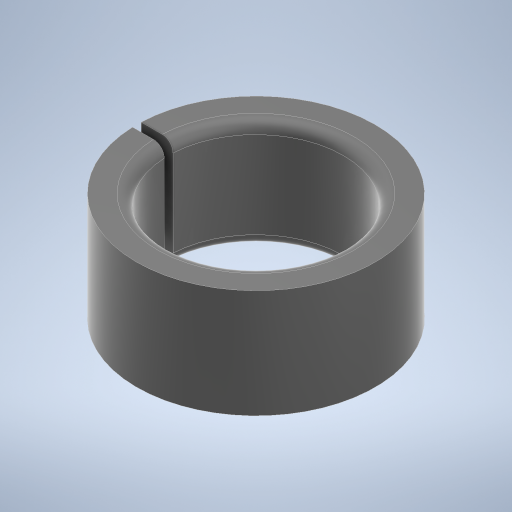
# Autodesk Inventor part: fittingRing
Saved by Autodesk Inventor 2023 (Build 270158000, 158)
## iProperties
Created: 2023-06-24
Part Number: fittingRing
Material: Пластик ПАЭК
Document SubType Name: Modeling
Designer: khrip
Density: 1.32 g/cm^3
Appearance: Гладкая — черная
Author: khrip
Autodesk Inventor part; units mm, degrees
ref_plane "YZ Plane" through (0, 0, 0) normal (1, 0, 0) x (0, 1, 0)
ref_plane "XZ Plane" through (0, 0, 0) normal (0, 1, 0) x (-1, 0, 0)
ref_plane "XY Plane" through (0, 0, 0) normal (0, 0, 1) x (1, 0, 0)
sketch "Эскиз1" plane through (0, 0, 0) normal (0, 1, 0) x (-1, 0, 0)
  circle A0 centre (0, 0) radius 4.0333
  circle A1 centre (0, 0) radius 5.5
  line L0 (-0.3176, 0.2) -> (8.3843, 0.2)
  line L1 (8.3843, 0.2) -> (8.3843, -0.2)
  line L2 (8.3843, -0.2) -> (-0.3176, -0.2)
  line L3 (-0.3176, -0.2) -> (-0.3176, 0.2)
  line L4 (-0.3176, 0.2) -> (8.3843, -0.2) construction
  line L5 (8.3843, 0.2) -> (-0.3176, -0.2) construction
  point P0 (4.0333, 0)
  point P1 (5.4964, -0.2)
  point P2 (4.0284, -0.2)
  point P3 (4.0284, 0.2)
  point P4 (5.4964, 0.2)
  dimension "d0" = 8.0667
  dimension "d1" = 11
  dimension "d2" = 0.4
  constraints: 12 end point, 2 coincident, 2 midpoint, 2 parallel, 1 centre point, 1 horizontal, 1 perpendicular, 3 other
  measures "d1" diameter of A1
  measures "d2" distance of L0.end L1.end
extrude "Выдавливание1" add sketch "Эскиз1" along normal blind 5 contours A0 L2 A1 L0 picked at (-4.9726, 0.1659)
fillet "Сопряжение1" radius 0.5 2 edges at (4.0333, 0, 0) (4.0333, 5, 0)
